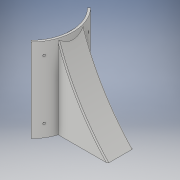
# Autodesk Inventor part: top camera cover
Saved by Autodesk Inventor 2017 (Build 210142000, 142)
## iProperties
Created: 2016-11-05
Part Number: top camera cover
Material: Generic
Document SubType Name: Modeling
Designer: Juan Maldonado
Density: 1 g/cm^3
Appearance: Default
Author: Juan Maldonado
Autodesk Inventor part; units mm, degrees
sketch "Sketch1" plane through (0, 0, 0) normal (0, 0, 1) x (1, 0, 0)
  line L0 (0, 0) -> (152.4, 0)
  line L1 (0, 0) -> (0, 254)
  arc A0 (0, 254) -> (152.4, 0) centre (642.353, 466.6918) ccw
  dimension "d0" = 152.4
  dimension "d1" = 254
  constraints: 4 end point, 2 point on circle, 1 centre point, 1 horizontal, 1 vertical
  measures "d0" distance of L0.start L0.end
  measures "d1" distance of L0.start L1.end
extrude "Extrusion1" add sketch "Sketch1" along normal blind 76.2
shell "Shell2" thickness 2.54 removed faces 1 at (0, 169.3333, 25.4)
sketch "Sketch10" plane through (0, 0, 0) normal (0, -1, 0) x (1, 0, 0)
  line L0 (0, 76.2) -> (152.4, 76.2) projected
  line L1 (0, 76.2) -> (152.4, 76.2)
  line L2 (152.4, 76.2) -> (152.4, 0)
  line L3 (152.4, 0) -> (0, 0)
  line L4 (0, 0) -> (0, 76.2)
  constraints: 8 end point, 2 parallel, 1 horizontal, 1 perpendicular
extrude "Extrusion6" cut sketch "Sketch10" against normal blind 2.54
ref_plane "Work Plane4" through (149.9931, 2.54, 38.1) normal (0, -1, 0) x (1, 0, 0)
sketch "Sketch11" plane through (149.9931, 2.54, 38.1) normal (0, -1, 0) x (1, 0, 0)
  arc A0 (-179.4346, -89.6601) -> (-179.4346, 88.4945) centre (-269.9566, -0.5828) ccw
  arc A1 (-184.1326, -85.3806) -> (-184.1326, 84.2151) centre (-269.9566, -0.5828) ccw
  line L0 (-184.1326, -85.3806) -> (-179.4346, -89.6601)
  line L1 (-184.1326, 84.2151) -> (-179.4346, 88.4945)
  point P0 (-149.9931, -38.1)
  dimension "d55" = 254
  dimension "d56" = 241.3
  constraints: 4 end point, 4 point on circle, 2 centre point, 1 coincident
  measures "d55" diameter of A0
  measures "d56" diameter of A1
extrude "Extrusion7" add sketch "Sketch11" against normal blind 251.46
ref_plane "Work Plane5" through (1.002, 2.54, 76.2) normal (0.9525, 0, 0.3046) x (0, 1, 0)
sketch "Sketch12" plane through (1.002, 2.54, 76.2) normal (0.9525, 0, 0.3046) x (0, 1, 0)
  circle A0 centre (214.2951, 31.3452) radius 3.175
  circle A1 centre (37.4631, 31.3452) radius 3.175
  point P0 (-2.54, -72.2741)
  dimension "d59" = 6.35
  dimension "d60" = 6.35
  constraints: 2 centre point
  measures "d59" diameter of A0
  measures "d60" diameter of A1
hole "Hole3" at (-8.5454, 216.8351, 106.0558) at (-8.5454, 40.0031, 106.0558) direction (-0.9525, 0, -0.3046) diameter 6.35 end through all
fillet "Fillet2" radius 3.175 2 edges at (62.0446, 118.7014, 76.2) (62.3397, 118.2097, 0)
ref_plane "Work Plane7" through (1.3685, 2.54, 0) normal (0.9554, 0, -0.2954) x (0, 1, 0)
sketch "Sketch14" plane through (1.3685, 2.54, 0) normal (0.9554, 0, -0.2954) x (0, 1, 0)
  circle A0 centre (211.1201, -28.0477) radius 3.175
  circle A1 centre (37.3894, -28.0477) radius 3.175
  point P0 (-2.54, -0.4043)
  dimension "d78" = 6.35
  dimension "d79" = 6.35
  constraints: 2 centre point
  measures "d78" diameter of A0
  measures "d79" diameter of A1
hole "Hole5" at (-6.9171, 39.9294, -26.7959) at (-6.9171, 213.6601, -26.7959) direction (-0.9554, 0, 0.2954) diameter 6.35 end through all
body "Solid1"
